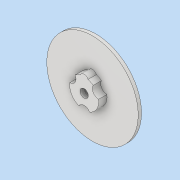
# Autodesk Inventor part: SpoolEndSpurSide
Saved by Autodesk Inventor 2017 (Build 210142000, 142)
## iProperties
Created: 2016-11-06
Part Number: SpoolEndSpurSide
Material: ABS Plastic
Document SubType Name: Modeling
Designer: techn
Density: 1.06 g/cm^3
Appearance: Smooth - White
Author: techn
Autodesk Inventor part; units mm, degrees
ref_plane "YZ Plane" through (0, 0, 0) normal (1, 0, 0) x (0, 1, 0)
ref_plane "XZ Plane" through (0, 0, 0) normal (0, 1, 0) x (-1, 0, 0)
ref_plane "XY Plane" through (0, 0, 0) normal (0, 0, 1) x (1, 0, 0)
sketch "Sketch1" plane through (0, 0, 0) normal (0, 0, 1) x (1, 0, 0)
  circle A0 centre (0, 0) radius 34.925
  dimension "d0" = 69.85
  constraints: 1 centre point, 1 coincident
  measures "d0" diameter of A0
extrude "Extrusion1" add sketch "Sketch1" along normal blind 2.54
sketch "Sketch2" plane through (0, 0, 2.54) normal (0, 0, 1) x (1, 0, 0)
  circle A0 centre (0, 0) radius 11.1125
  line L0 (0, 0) -> (0, -12.7)
  circle A1 centre (0, -12.7) radius 4.7625
  circle A2 centre (10.9985, 6.35) radius 4.7625
  circle A3 centre (-10.9985, 6.35) radius 4.7625
  dimension "d3" = 22.225
  dimension "d4" = 12.7
  dimension "d5" = 9.525
  dimension "d8" = 360
  constraints: 4 centre point, 2 coincident, 2 end point, 1 vertical, 7 other
  measures "d3" diameter of A0
  measures "d4" distance of L0.start L0.end
  measures "d5" diameter of A1
extrude "Extrusion2" add sketch "Sketch2" along normal blind 6.35 contours A0 A1 A3 A2 | A2 A0 | A0 L0 A1 | A0 A1 L0 | A3 A0 picked at (9.3538, 3.9651) picked at (-8.1265, 6.0404)
extrude "Extrusion3" cut sketch "Sketch2" along normal blind 6.35 contours A2 A0 | A0 A2 | A1 A0 | A0 L0 A1 | A0 A1 L0 | A3 A0 | A0 A3
sketch "Sketch3" plane through (0, 0, 2.54) normal (0, 0, 1) x (1, 0, 0)
  line L0 (0, 0) -> (0, 9.525)
  circle A0 centre (0, 9.525) radius 3.175
  dimension "d14" = 9.525
  dimension "d15" = 6.35
  constraints: 2 end point, 1 centre point, 1 coincident, 1 vertical
  measures "d14" distance of L0.start L0.end
  measures "d15" diameter of A0
extrude "Extrusion4" add sketch "Sketch3" along normal blind 6.35
sketch "Sketch4" plane through (0, 0, 8.89) normal (0, 0, 1) x (1, 0, 0)
  circle A0 centre (0, 0) radius 3.175
  circle A1 centre (0, 0) radius 2.3813
  dimension "d18" = 6.35
  dimension "d19" = 4.7625
  constraints: 2 centre point, 2 coincident
  measures "d18" diameter of A0
  measures "d19" diameter of A1
extrude "Extrusion5" cut sketch "Sketch4" against normal blind 3.175 contours A0 | A1
extrude "Extrusion6" cut sketch "Sketch4" against normal through all contours A1
body "Solid1"
